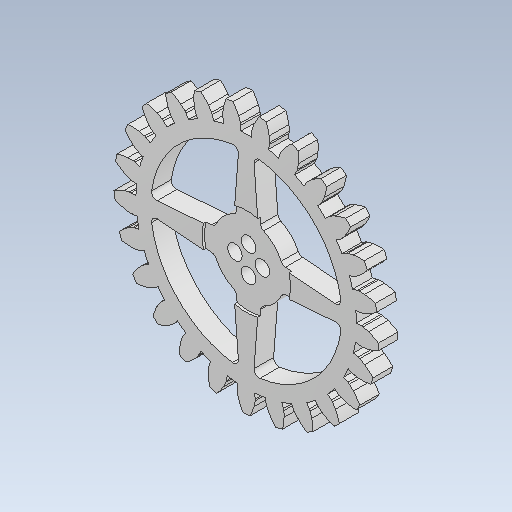
# Autodesk Inventor part: ｍ2歯数25ギアネジ
Saved by Autodesk Inventor 2020.2 (Build 242310000, 310)
## iProperties
Created: 2020-04-14
Part Number: ｍ2歯数25ギアネジ
Material: アルミニウム 2014-T4
Document SubType Name: Modeling
Designer: aoyama
Density: 2.8 g/cm^3
Appearance: サテン
Author: aoyama
Autodesk Inventor part; units mm, degrees
ref_plane "YZ Plane" through (0, 0, 0) normal (1, 0, 0) x (0, 1, 0)
ref_plane "XZ Plane" through (0, 0, 0) normal (0, 1, 0) x (-1, 0, 0)
ref_plane "XY Plane" through (0, 0, 0) normal (0, 0, 1) x (1, 0, 0)
sketch "スケッチ1" plane through (0, 0, 0) normal (0, 0, 1) x (1, 0, 0)
  arc A0 (-5.045, 28.8847) -> (-5.1025, 28.5361) centre (-2.8234, 28.3389) ccw
  arc A1 (-4.679, 29.9735) -> (-5.045, 28.8847) centre (1.0751, 27.4336) ccw
  arc A2 (-3.5593, 31.9385) -> (-4.679, 29.9735) centre (5.2754, 25.6027) ccw
  arc A3 (-7.3535, 28.5361) -> (-7.4111, 28.8847) centre (-9.6326, 28.3389) ccw
  arc A4 (-7.4111, 28.8847) -> (-7.777, 29.9735) centre (-13.5311, 27.4336) ccw
  arc A5 (-7.777, 29.9735) -> (-8.8968, 31.9385) centre (-17.7315, 25.6027) ccw
  arc A6 (-5.1501, 27.5449) -> (-7.306, 27.5449) centre (-6.228, 5.0707) ccw
  arc A7 (-8.8968, 31.9385) -> (-10.3249, 31.7581) centre (-6.228, 5.0707) ccw
  line L0 (-5.1501, 27.5449) -> (-5.1025, 28.5361)
  line L1 (-7.306, 27.5449) -> (-7.3535, 28.5361)
  arc A8 (-15.4947, 30.4307) -> (-16.8331, 29.9008) centre (-6.228, 5.0707) ccw
  arc A9 (-13.9214, 28.8059) -> (-15.4947, 30.4307) centre (-22.4762, 22.0969) ccw
  arc A10 (-13.2962, 27.8424) -> (-13.9214, 28.8059) centre (-18.8631, 24.9148) ccw
  line L2 (-12.8612, 26.5708) -> (-13.1538, 27.519)
  arc A11 (-13.1538, 27.519) -> (-13.2962, 27.8424) centre (-15.3122, 26.7612) ccw
  arc A12 (-11.0044, 28.4308) -> (-10.9735, 28.0788) centre (-8.7169, 28.4546) ccw
  arc A13 (-10.773, 27.1069) -> (-12.8612, 26.5708) centre (-6.228, 5.0707) ccw
  arc A14 (-10.9208, 29.5763) -> (-11.0044, 28.4308) centre (-4.7158, 28.5472) ccw
  arc A15 (-10.3249, 31.7581) -> (-10.9208, 29.5763) centre (-0.1921, 27.8185) ccw
  line L3 (-10.773, 27.1069) -> (-10.9735, 28.0788)
  arc A16 (-21.5103, 27.3295) -> (-22.6749, 26.4834) centre (-6.228, 5.0707) ccw
  arc A17 (-19.5824, 26.1469) -> (-21.5103, 27.3295) centre (-26.1999, 17.5212) ccw
  arc A18 (-18.7372, 25.3692) -> (-19.5824, 26.1469) centre (-23.4012, 21.1491) ccw
  line L4 (-17.9997, 24.2457) -> (-18.5188, 25.0914)
  arc A19 (-18.5188, 25.0914) -> (-18.7372, 25.3692) centre (-20.421, 23.8206) ccw
  arc A20 (-16.6638, 26.509) -> (-16.5463, 26.1758) centre (-14.4541, 27.101) ccw
  arc A21 (-16.1104, 25.2843) -> (-17.9997, 24.2457) centre (-6.228, 5.0707) ccw
  arc A22 (-16.8676, 27.6394) -> (-16.6638, 26.509) centre (-10.6017, 28.1857) ccw
  arc A23 (-16.8331, 29.9008) -> (-16.8676, 27.6394) centre (-6.0388, 28.6049) ccw
  line L5 (-16.1104, 25.2843) -> (-16.5463, 26.1758)
  arc A24 (-26.5657, 22.8296) -> (-27.4833, 21.7205) centre (-6.228, 5.0707) ccw
  arc A25 (-24.4043, 22.1637) -> (-26.5657, 22.8296) centre (-28.6688, 12.1633) ccw
  arc A26 (-23.3922, 21.6205) -> (-24.4043, 22.1637) centre (-26.8602, 16.3732) ccw
  line L6 (-22.3984, 20.7158) -> (-23.1116, 21.4058)
  arc A27 (-23.1116, 21.4058) -> (-23.3922, 21.6205) centre (-24.638, 19.7019) ccw
  arc A28 (-21.6674, 23.2402) -> (-21.4707, 22.9467) centre (-19.6743, 24.3631) ccw
  arc A29 (-20.8269, 22.1916) -> (-22.3984, 20.7158) centre (-6.228, 5.0707) ccw
  arc A30 (-22.146, 24.2844) -> (-21.6674, 23.2402) centre (-16.2127, 26.3719) ccw
  arc A31 (-22.6749, 26.4834) -> (-22.146, 24.2844) centre (-11.8975, 27.9126) ccw
  line L7 (-20.8269, 22.1916) -> (-21.4707, 22.9467)
  arc A32 (-30.3432, 17.2139) -> (-30.9561, 15.9115) centre (-6.228, 5.0707) ccw
  arc A33 (-28.0841, 17.1064) -> (-30.3432, 17.2139) centre (-29.7276, 6.3596) ccw
  arc A34 (-26.9688, 16.832) -> (-28.0841, 17.1064) centre (-29.0228, 10.8871) ccw
  line L8 (-25.7812, 16.2029) -> (-26.6435, 16.6938)
  arc A35 (-26.6435, 16.6938) -> (-26.9688, 16.832) centre (-27.6983, 14.6638) ccw
  arc A36 (-25.7009, 18.8298) -> (-25.4374, 18.5944) centre (-24.0497, 20.4131) ccw
  arc A37 (-24.626, 18.0232) -> (-25.7812, 16.2029) centre (-6.228, 5.0707) ccw
  arc A38 (-26.4241, 19.7222) -> (-25.7009, 18.8298) centre (-21.1964, 23.2196) ccw
  arc A39 (-27.4833, 21.7205) -> (-26.4241, 19.7222) centre (-17.3999, 25.785) ccw
  line L9 (-24.626, 18.0232) -> (-25.4374, 18.5944)
  arc A40 (-32.6055, 10.8352) -> (-32.8752, 9.4213) centre (-6.228, 5.0707) ccw
  arc A41 (-30.3906, 11.2929) -> (-32.6055, 10.8352) centre (-29.3099, 0.475) ccw
  arc A42 (-29.2421, 11.3045) -> (-30.3906, 11.2929) centre (-29.7531, 5.0356) ccw
  line L10 (-27.9353, 10.9904) -> (-28.8927, 11.2515)
  arc A43 (-28.8927, 11.2515) -> (-29.2421, 11.3045) centre (-29.4094, 9.023) ccw
  arc A44 (-28.5109, 13.5548) -> (-28.1971, 13.3923) centre (-27.3053, 15.499) ccw
  arc A45 (-27.2691, 13.0408) -> (-27.9353, 10.9904) centre (-6.228, 5.0707) ccw
  arc A46 (-29.4333, 14.2393) -> (-28.5109, 13.5548) centre (-25.2396, 18.9269) ccw
  arc A47 (-30.9561, 15.9115) -> (-29.4333, 14.2393) centre (-22.2003, 22.3559) ccw
  line L11 (-27.2691, 13.0408) -> (-28.1971, 13.3923)
  arc A48 (-33.2104, 4.0943) -> (-33.12, 2.6577) centre (-6.228, 5.0707) ccw
  arc A49 (-31.1789, 5.0885) -> (-33.2104, 4.0943) centre (-27.4418, -5.1208) ccw
  arc A50 (-30.0693, 5.3853) -> (-31.1789, 5.0885) centre (-29.0053, -0.8138) ccw
  line L12 (-28.7255, 5.4061) -> (-29.7177, 5.4209)
  arc A51 (-29.7177, 5.4209) -> (-30.0693, 5.3853) centre (-29.664, 3.1339) ccw
  arc A52 (-29.9207, 7.7468) -> (-29.5764, 7.6674) centre (-29.2365, 9.9297) ccw
  arc A53 (-28.5902, 7.5577) -> (-28.7255, 5.4061) centre (-6.228, 5.0707) ccw
  arc A54 (-30.9844, 8.1803) -> (-29.9207, 7.7468) centre (-28.0882, 13.7636) ccw
  arc A55 (-32.8752, 9.4213) -> (-30.9844, 8.1803) centre (-25.9972, 17.8407) ccw
  line L13 (-28.5902, 7.5577) -> (-29.5764, 7.6674)
  arc A56 (-32.1198, -2.5852) -> (-31.675, -3.9543) centre (-6.228, 5.0707) ccw
  arc A57 (-30.3994, -1.1171) -> (-32.1198, -2.5852) centre (-24.2408, -10.0763) ccw
  arc A58 (-29.3985, -0.5536) -> (-30.3994, -1.1171) centre (-26.8263, -6.2934) ccw
  line L14 (-28.1021, -0.1994) -> (-29.0668, -0.4318)
  arc A59 (-29.0668, -0.4318) -> (-29.3985, -0.5536) centre (-28.4461, -2.6336) ccw
  arc A60 (-29.8419, 1.7705) -> (-29.4886, 1.7793) centre (-29.722, 4.055) ccw
  arc A61 (-28.5061, 1.9184) -> (-28.1021, -0.1994) centre (-6.228, 5.0707) ccw
  arc A62 (-30.9799, 1.926) -> (-29.8419, 1.7705) centre (-29.5632, 8.0541) ccw
  arc A63 (-33.12, 2.6577) -> (-30.9799, 1.926) centre (-28.5519, 12.5231) ccw
  line L15 (-28.5061, 1.9184) -> (-29.4886, 1.7793)
  arc A64 (-29.4024, -8.7837) -> (-28.6311, -9.9991) centre (-6.228, 5.0707) ccw
  arc A65 (-28.1012, -6.9339) -> (-29.4024, -8.7837) centre (-19.908, -14.08) ccw
  arc A66 (-27.2718, -6.1392) -> (-28.1012, -6.9339) centre (-23.353, -11.0589) ccw
  line L16 (-26.1043, -5.4737) -> (-26.9809, -5.9387)
  arc A67 (-26.9809, -5.9387) -> (-27.2718, -6.1392) centre (-25.8321, -7.9169) ccw
  arc A68 (-28.2793, -3.9983) -> (-27.9393, -3.9019) centre (-28.7313, -1.7558) ccw
  arc A69 (-27.0222, -3.5229) -> (-26.1043, -5.4737) centre (-6.228, 5.0707) ccw
  arc A70 (-29.4202, -4.1308) -> (-28.2793, -3.9983) centre (-29.572, 2.1572) ccw
  arc A71 (-31.675, -3.9543) -> (-29.4202, -4.1308) centre (-29.7038, 6.7373) ccw
  line L17 (-27.0222, -3.5229) -> (-27.9393, -3.9019)
  arc A72 (-25.2289, -14.1117) -> (-24.1796, -15.0971) centre (-6.228, 5.0707) ccw
  arc A73 (-24.4285, -11.9964) -> (-25.2289, -14.1117) centre (-14.7156, -16.8804) ccw
  arc A74 (-23.8229, -11.0204) -> (-24.4285, -11.9964) centre (-18.8037, -14.811) ccw
  line L18 (-22.8576, -10.0854) -> (-23.591, -10.7538)
  arc A75 (-23.591, -10.7538) -> (-23.8229, -11.0204) centre (-21.9863, -12.3842) ccw
  arc A76 (-25.3311, -9.1973) -> (-25.0258, -9.0194) centre (-26.3266, -7.1376) ccw
  arc A77 (-24.2318, -8.4242) -> (-22.8576, -10.0854) centre (-6.228, 5.0707) ccw
  arc A78 (-26.4033, -9.6093) -> (-25.3311, -9.1973) centre (-28.1141, -3.5567) ccw
  arc A79 (-28.6311, -9.9991) -> (-26.4033, -9.6093) centre (-29.3808, 0.8467) ccw
  line L19 (-24.2318, -8.4242) -> (-25.0258, -9.0194)
  arc A80 (-19.8615, -18.2344) -> (-18.6, -18.9279) centre (-6.228, 5.0707) ccw
  arc A81 (-19.6123, -15.9865) -> (-19.8615, -18.2344) centre (-8.9899, -18.3015) ccw
  arc A82 (-19.2684, -14.8906) -> (-19.6123, -15.9865) centre (-13.4642, -17.3138) ccw
  line L20 (-18.5659, -13.7448) -> (-19.1101, -14.5747)
  arc A83 (-19.1101, -14.5747) -> (-19.2684, -14.8906) centre (-17.1503, -15.7548) ccw
  arc A84 (-21.1826, -13.4998) -> (-20.9312, -13.2516) centre (-22.6591, -11.7524) ccw
  arc A85 (-20.3101, -12.4776) -> (-18.5659, -13.7448) centre (-6.228, 5.0707) ccw
  arc A86 (-22.1186, -14.1655) -> (-21.1826, -13.4998) centre (-25.2809, -8.7285) ccw
  arc A87 (-24.1796, -15.0971) -> (-22.1186, -14.1655) centre (-27.6029, -4.7784) ccw
  line L21 (-20.3101, -12.4776) -> (-20.9312, -13.2516)
  arc A88 (-13.6374, -20.8927) -> (-12.2431, -21.2507) centre (-6.228, 5.0707) ccw
  arc A89 (-13.9551, -18.6534) -> (-13.6374, -20.8927) centre (-3.0907, -18.2541) ccw
  arc A90 (-13.8946, -17.5064) -> (-13.9551, -18.6534) centre (-7.6701, -18.4101) ccw
  line L22 (-13.4991, -16.222) -> (-13.8197, -17.1611)
  arc A91 (-13.8197, -17.1611) -> (-13.8946, -17.5064) centre (-11.6281, -17.8168) ccw
  arc A92 (-16.0945, -16.6354) -> (-15.9127, -16.3325) centre (-17.9591, -15.3101) ccw
  arc A93 (-15.5036, -15.4284) -> (-13.4991, -16.222) centre (-6.228, 5.0707) ccw
  arc A94 (-16.8356, -17.513) -> (-16.0945, -16.6354) centre (-21.2506, -13.0332) ccw
  arc A95 (-18.6, -18.9279) -> (-16.8356, -17.513) centre (-24.482, -9.7847) ccw
  line L23 (-15.5036, -15.4284) -> (-15.9127, -16.3325)
  arc A96 (-6.9478, -21.9197) -> (-5.5083, -21.9197) centre (-6.228, 5.0707) ccw
  arc A97 (-7.8124, -19.8298) -> (-6.9478, -21.9197) centre (2.6114, -16.7411) ccw
  arc A98 (-8.039, -18.7037) -> (-7.8124, -19.8298) centre (-1.7853, -18.0311) ccw
  line L24 (-7.9753, -17.3613) -> (-8.0524, -18.3506)
  arc A99 (-8.0524, -18.3506) -> (-8.039, -18.7037) centre (-5.7665, -18.4406) ccw
  arc A100 (-10.3864, -18.4072) -> (-10.2856, -18.0685) centre (-12.5221, -17.5872) ccw
  arc A101 (-10.1142, -17.0911) -> (-7.9753, -17.3613) centre (-6.228, 5.0707) ccw
  arc A102 (-10.8859, -19.4415) -> (-10.3864, -18.4072) centre (-16.2763, -16.2004) ccw
  arc A103 (-12.2431, -21.2507) -> (-10.8859, -19.4415) centre (-20.2141, -13.8576) ccw
  line L25 (-10.1142, -17.0911) -> (-10.2856, -18.0685)
  arc A104 (-0.2129, -21.2507) -> (1.1813, -20.8927) centre (-6.228, 5.0707) ccw
  arc A105 (-1.5701, -19.4415) -> (-0.2129, -21.2507) centre (7.758, -13.8576) ccw
  arc A106 (-2.0696, -18.4072) -> (-1.5701, -19.4415) centre (3.8203, -16.2004) ccw
  line L26 (-2.3418, -17.0911) -> (-2.1704, -18.0685)
  arc A107 (-2.1704, -18.0685) -> (-2.0696, -18.4072) centre (0.066, -17.5872) ccw
  arc A108 (-4.4171, -18.7037) -> (-4.4037, -18.3506) centre (-6.6895, -18.4406) ccw
  arc A109 (-4.4807, -17.3613) -> (-2.3418, -17.0911) centre (-6.228, 5.0707) ccw
  arc A110 (-4.6437, -19.8298) -> (-4.4171, -18.7037) centre (-10.6707, -18.0311) ccw
  arc A111 (-5.5083, -21.9197) -> (-4.6437, -19.8298) centre (-15.0674, -16.7411) ccw
  line L27 (-4.4807, -17.3613) -> (-4.4037, -18.3506)
  arc A112 (6.144, -18.9279) -> (7.4054, -18.2344) centre (-6.228, 5.0707) ccw
  arc A113 (4.3795, -17.513) -> (6.144, -18.9279) centre (12.0259, -9.7847) ccw
  arc A114 (3.6385, -16.6354) -> (4.3795, -17.513) centre (8.7945, -13.0332) ccw
  line L28 (3.0475, -15.4284) -> (3.4566, -16.3325)
  arc A115 (3.4566, -16.3325) -> (3.6385, -16.6354) centre (5.5031, -15.3101) ccw
  arc A116 (1.4385, -17.5064) -> (1.3637, -17.1611) centre (-0.828, -17.8168) ccw
  arc A117 (1.043, -16.222) -> (3.0475, -15.4284) centre (-6.228, 5.0707) ccw
  arc A118 (1.4991, -18.6534) -> (1.4385, -17.5064) centre (-4.786, -18.4101) ccw
  arc A119 (1.1813, -20.8927) -> (1.4991, -18.6534) centre (-9.3653, -18.2541) ccw
  line L29 (1.043, -16.222) -> (1.3637, -17.1611)
  arc A120 (11.7235, -15.0971) -> (12.7728, -14.1117) centre (-6.228, 5.0707) ccw
  arc A121 (9.6626, -14.1655) -> (11.7235, -15.0971) centre (15.1468, -4.7784) ccw
  arc A122 (8.7266, -13.4998) -> (9.6626, -14.1655) centre (12.8248, -8.7285) ccw
  line L30 (7.854, -12.4776) -> (8.4751, -13.2516)
  arc A123 (8.4751, -13.2516) -> (8.7266, -13.4998) centre (10.203, -11.7524) ccw
  arc A124 (6.8124, -14.8906) -> (6.654, -14.5747) centre (4.6943, -15.7548) ccw
  arc A125 (6.1099, -13.7448) -> (7.854, -12.4776) centre (-6.228, 5.0707) ccw
  arc A126 (7.1563, -15.9865) -> (6.8124, -14.8906) centre (1.0082, -17.3138) ccw
  arc A127 (7.4054, -18.2344) -> (7.1563, -15.9865) centre (-3.4661, -18.3015) ccw
  line L31 (6.1099, -13.7448) -> (6.654, -14.5747)
  arc A128 (16.1751, -9.9991) -> (16.9464, -8.7837) centre (-6.228, 5.0707) ccw
  arc A129 (13.9472, -9.6093) -> (16.1751, -9.9991) centre (16.9247, 0.8467) ccw
  arc A130 (12.8751, -9.1973) -> (13.9472, -9.6093) centre (15.658, -3.5567) ccw
  line L32 (11.7757, -8.4242) -> (12.5697, -9.0194)
  arc A131 (12.5697, -9.0194) -> (12.8751, -9.1973) centre (13.8706, -7.1376) ccw
  arc A132 (11.3669, -11.0204) -> (11.1349, -10.7538) centre (9.5302, -12.3842) ccw
  arc A133 (10.4015, -10.0854) -> (11.7757, -8.4242) centre (-6.228, 5.0707) ccw
  arc A134 (11.9725, -11.9964) -> (11.3669, -11.0204) centre (6.3477, -14.811) ccw
  arc A135 (12.7728, -14.1117) -> (11.9725, -11.9964) centre (2.2596, -16.8804) ccw
  line L33 (10.4015, -10.0854) -> (11.1349, -10.7538)
  arc A136 (19.219, -3.9543) -> (19.6638, -2.5852) centre (-6.228, 5.0707) ccw
  arc A137 (16.9642, -4.1308) -> (19.219, -3.9543) centre (17.2478, 6.7373) ccw
  arc A138 (15.8232, -3.9983) -> (16.9642, -4.1308) centre (17.116, 2.1572) ccw
  line L34 (14.5662, -3.5229) -> (15.4833, -3.9019)
  arc A139 (15.4833, -3.9019) -> (15.8232, -3.9983) centre (16.2752, -1.7558) ccw
  arc A140 (14.8158, -6.1392) -> (14.5248, -5.9387) centre (13.376, -7.9169) ccw
  arc A141 (13.6482, -5.4737) -> (14.5662, -3.5229) centre (-6.228, 5.0707) ccw
  arc A142 (15.6451, -6.9339) -> (14.8158, -6.1392) centre (10.897, -11.0589) ccw
  arc A143 (16.9464, -8.7837) -> (15.6451, -6.9339) centre (7.4519, -14.08) ccw
  line L35 (13.6482, -5.4737) -> (14.5248, -5.9387)
  arc A144 (20.6639, 2.6577) -> (20.7543, 4.0943) centre (-6.228, 5.0707) ccw
  arc A145 (18.5239, 1.926) -> (20.6639, 2.6577) centre (16.0958, 12.5231) ccw
  arc A146 (17.3858, 1.7705) -> (18.5239, 1.926) centre (17.1072, 8.0541) ccw
  line L36 (16.05, 1.9184) -> (17.0326, 1.7793)
  arc A147 (17.0326, 1.7793) -> (17.3858, 1.7705) centre (17.2659, 4.055) ccw
  arc A148 (16.9425, -0.5536) -> (16.6108, -0.4318) centre (15.99, -2.6336) ccw
  arc A149 (15.6461, -0.1994) -> (16.05, 1.9184) centre (-6.228, 5.0707) ccw
  arc A150 (17.9433, -1.1171) -> (16.9425, -0.5536) centre (14.3702, -6.2934) ccw
  arc A151 (19.6638, -2.5852) -> (17.9433, -1.1171) centre (11.7847, -10.0763) ccw
  line L37 (15.6461, -0.1994) -> (16.6108, -0.4318)
  arc A152 (20.4192, 9.4213) -> (20.1494, 10.8352) centre (-6.228, 5.0707) ccw
  arc A153 (18.5283, 8.1803) -> (20.4192, 9.4213) centre (13.5411, 17.8407) ccw
  arc A154 (17.4647, 7.7468) -> (18.5283, 8.1803) centre (15.6321, 13.7636) ccw
  line L38 (16.1341, 7.5577) -> (17.1203, 7.6674)
  arc A155 (17.1203, 7.6674) -> (17.4647, 7.7468) centre (16.7804, 9.9297) ccw
  arc A156 (17.6132, 5.3853) -> (17.2617, 5.4209) centre (17.208, 3.1339) ccw
  arc A157 (16.2695, 5.4061) -> (16.1341, 7.5577) centre (-6.228, 5.0707) ccw
  arc A158 (18.7228, 5.0885) -> (17.6132, 5.3853) centre (16.5492, -0.8138) ccw
  arc A159 (20.7543, 4.0943) -> (18.7228, 5.0885) centre (14.9857, -5.1208) ccw
  line L39 (16.2695, 5.4061) -> (17.2617, 5.4209)
  arc A160 (18.5001, 15.9115) -> (17.8872, 17.2139) centre (-6.228, 5.0707) ccw
  arc A161 (16.9772, 14.2393) -> (18.5001, 15.9115) centre (9.7443, 22.3559) ccw
  arc A162 (16.0548, 13.5548) -> (16.9772, 14.2393) centre (12.7835, 18.9269) ccw
  line L40 (14.8131, 13.0408) -> (15.741, 13.3923)
  arc A163 (15.741, 13.3923) -> (16.0548, 13.5548) centre (14.8492, 15.499) ccw
  arc A164 (16.786, 11.3045) -> (16.4366, 11.2515) centre (16.9534, 9.023) ccw
  arc A165 (15.4793, 10.9904) -> (14.8131, 13.0408) centre (-6.228, 5.0707) ccw
  arc A166 (17.9345, 11.2929) -> (16.786, 11.3045) centre (17.2971, 5.0356) ccw
  arc A167 (20.1494, 10.8352) -> (17.9345, 11.2929) centre (16.8538, 0.475) ccw
  line L41 (15.4793, 10.9904) -> (16.4366, 11.2515)
  arc A168 (15.0272, 21.7205) -> (14.1097, 22.8296) centre (-6.228, 5.0707) ccw
  arc A169 (13.968, 19.7222) -> (15.0272, 21.7205) centre (4.9438, 25.785) ccw
  arc A170 (13.2449, 18.8298) -> (13.968, 19.7222) centre (8.7403, 23.2196) ccw
  line L42 (12.1699, 18.0232) -> (12.9813, 18.5944)
  arc A171 (12.9813, 18.5944) -> (13.2449, 18.8298) centre (11.5936, 20.4131) ccw
  arc A172 (14.5127, 16.832) -> (14.1875, 16.6938) centre (15.2422, 14.6638) ccw
  arc A173 (13.3251, 16.2029) -> (12.1699, 18.0232) centre (-6.228, 5.0707) ccw
  arc A174 (15.628, 17.1064) -> (14.5127, 16.832) centre (16.5667, 10.8871) ccw
  arc A175 (17.8872, 17.2139) -> (15.628, 17.1064) centre (17.2715, 6.3596) ccw
  line L43 (13.3251, 16.2029) -> (14.1875, 16.6938)
  arc A176 (10.2188, 26.4834) -> (9.0543, 27.3295) centre (-6.228, 5.0707) ccw
  arc A177 (9.6899, 24.2844) -> (10.2188, 26.4834) centre (-0.5586, 27.9126) ccw
  arc A178 (9.2114, 23.2402) -> (9.6899, 24.2844) centre (3.7567, 26.3719) ccw
  line L44 (8.3708, 22.1916) -> (9.0146, 22.9467)
  arc A179 (9.0146, 22.9467) -> (9.2114, 23.2402) centre (7.2183, 24.3631) ccw
  arc A180 (10.9362, 21.6205) -> (10.6556, 21.4058) centre (12.182, 19.7019) ccw
  arc A181 (9.9424, 20.7158) -> (8.3708, 22.1916) centre (-6.228, 5.0707) ccw
  arc A182 (11.9482, 22.1637) -> (10.9362, 21.6205) centre (14.4041, 16.3732) ccw
  arc A183 (14.1097, 22.8296) -> (11.9482, 22.1637) centre (16.2127, 12.1633) ccw
  line L45 (9.9424, 20.7158) -> (10.6556, 21.4058)
  arc A184 (4.377, 29.9008) -> (3.0386, 30.4307) centre (-6.228, 5.0707) ccw
  arc A185 (4.4116, 27.6394) -> (4.377, 29.9008) centre (-6.4172, 28.6049) ccw
  arc A186 (4.2077, 26.509) -> (4.4116, 27.6394) centre (-1.8544, 28.1857) ccw
  line L46 (3.6544, 25.2843) -> (4.0902, 26.1758)
  arc A187 (4.0902, 26.1758) -> (4.2077, 26.509) centre (1.998, 27.101) ccw
  arc A188 (6.2812, 25.3692) -> (6.0628, 25.0914) centre (7.965, 23.8206) ccw
  arc A189 (5.5436, 24.2457) -> (3.6544, 25.2843) centre (-6.228, 5.0707) ccw
  arc A190 (7.1263, 26.1469) -> (6.2812, 25.3692) centre (10.9451, 21.1491) ccw
  arc A191 (9.0543, 27.3295) -> (7.1263, 26.1469) centre (13.7439, 17.5212) ccw
  line L47 (5.5436, 24.2457) -> (6.0628, 25.0914)
  arc A192 (-2.1312, 31.7581) -> (-3.5593, 31.9385) centre (-6.228, 5.0707) ccw
  arc A193 (-1.5353, 29.5763) -> (-2.1312, 31.7581) centre (-12.264, 27.8185) ccw
  arc A194 (-1.4516, 28.4308) -> (-1.5353, 29.5763) centre (-7.7403, 28.5472) ccw
  line L48 (-1.683, 27.1069) -> (-1.4826, 28.0788)
  arc A195 (-1.4826, 28.0788) -> (-1.4516, 28.4308) centre (-3.7391, 28.4546) ccw
  arc A196 (0.8402, 27.8424) -> (0.6977, 27.519) centre (2.8562, 26.7612) ccw
  arc A197 (0.4052, 26.5708) -> (-1.683, 27.1069) centre (-6.228, 5.0707) ccw
  arc A198 (1.4654, 28.8059) -> (0.8402, 27.8424) centre (6.407, 24.9148) ccw
  arc A199 (3.0386, 30.4307) -> (1.4654, 28.8059) centre (10.0201, 22.0969) ccw
  line L49 (0.4052, 26.5708) -> (0.6977, 27.519)
  line L50 (-6.228, 5.0707) -> (-6.228, 7.8707) construction
  circle A200 centre (-6.228, 7.8707) radius 2.8 construction
  circle A201 centre (-9.028, 5.0707) radius 2.8 construction
  circle A202 centre (-6.228, 2.2707) radius 2.8 construction
  circle A203 centre (-3.428, 5.0707) radius 2.8 construction
  circle A204 centre (-6.228, 7.8707) radius 1.5
  circle A205 centre (-9.028, 5.0707) radius 1.5
  circle A206 centre (-6.228, 2.2707) radius 1.5
  circle A207 centre (-3.428, 5.0707) radius 1.5
  point P0 (0, 0)
  point P1 (3.4566, -16.3325)
  point P2 (3.6385, -16.6354)
  point P3 (4.3795, -17.513)
  point P4 (6.144, -18.9279)
  point P5 (7.4054, -18.2344)
  point P6 (7.1563, -15.9865)
  point P7 (6.8124, -14.8906)
  point P8 (7.854, -12.4776)
  point P9 (8.4751, -13.2516)
  point P10 (8.7266, -13.4998)
  point P11 (9.6626, -14.1655)
  point P12 (11.7235, -15.0971)
  point P13 (12.7728, -14.1117)
  point P14 (11.9725, -11.9964)
  point P15 (11.3669, -11.0204)
  point P16 (11.7757, -8.4242)
  point P17 (12.5697, -9.0194)
  point P18 (12.8751, -9.1973)
  point P19 (13.9472, -9.6093)
  point P20 (16.1751, -9.9991)
  point P21 (16.9464, -8.7837)
  point P22 (15.6451, -6.9339)
  point P23 (14.8158, -6.1392)
  point P24 (14.5662, -3.5229)
  point P25 (15.4833, -3.9019)
  point P26 (15.8232, -3.9983)
  point P27 (16.9642, -4.1308)
  point P28 (19.219, -3.9543)
  point P29 (19.6638, -2.5852)
  point P30 (17.9433, -1.1171)
  point P31 (16.9425, -0.5536)
  point P32 (16.05, 1.9184)
  point P33 (17.0326, 1.7793)
  point P34 (17.3858, 1.7705)
  point P35 (18.5239, 1.926)
  point P36 (20.6639, 2.6577)
  point P37 (20.7543, 4.0943)
  point P38 (18.7228, 5.0885)
  point P39 (17.6132, 5.3853)
  point P40 (16.1341, 7.5577)
  point P41 (17.1203, 7.6674)
  point P42 (17.4647, 7.7468)
  point P43 (18.5283, 8.1803)
  point P44 (20.4192, 9.4213)
  point P45 (20.1494, 10.8352)
  point P46 (17.9345, 11.2929)
  point P47 (16.786, 11.3045)
  point P48 (14.8131, 13.0408)
  point P49 (15.741, 13.3923)
  point P50 (16.0548, 13.5548)
  point P51 (16.9772, 14.2393)
  point P52 (18.5001, 15.9115)
  point P53 (17.8872, 17.2139)
  point P54 (15.628, 17.1064)
  point P55 (14.5127, 16.832)
  point P56 (12.1699, 18.0232)
  point P57 (12.9813, 18.5944)
  point P58 (13.2449, 18.8298)
  point P59 (13.968, 19.7222)
  point P60 (15.0272, 21.7205)
  point P61 (14.1097, 22.8296)
  point P62 (11.9482, 22.1637)
  point P63 (10.9362, 21.6205)
  point P64 (8.3708, 22.1916)
  point P65 (9.0146, 22.9467)
  point P66 (9.2114, 23.2402)
  point P67 (9.6899, 24.2844)
  point P68 (10.2188, 26.4834)
  point P69 (9.0543, 27.3295)
  point P70 (7.1263, 26.1469)
  point P71 (6.2812, 25.3692)
  point P72 (3.6544, 25.2843)
  point P73 (4.0902, 26.1758)
  point P74 (4.2077, 26.509)
  point P75 (4.4116, 27.6394)
  point P76 (4.377, 29.9008)
  point P77 (3.0386, 30.4307)
  point P78 (1.4654, 28.8059)
  point P79 (0.8402, 27.8424)
  point P80 (-1.683, 27.1069)
  point P81 (-1.4826, 28.0788)
  point P82 (-1.4516, 28.4308)
  point P83 (-1.5353, 29.5763)
  point P84 (-2.1312, 31.7581)
  point P85 (-3.5593, 31.9385)
  point P86 (-4.679, 29.9735)
  point P87 (-5.045, 28.8847)
  point P88 (-7.4111, 28.8847)
  point P89 (-7.777, 29.9735)
  point P90 (-8.8968, 31.9385)
  point P91 (-10.3249, 31.7581)
  point P92 (-10.9208, 29.5763)
  point P93 (-11.0044, 28.4308)
  point P94 (-12.8612, 26.5708)
  point P95 (-13.1538, 27.519)
  point P96 (-13.2962, 27.8424)
  point P97 (-13.9214, 28.8059)
  point P98 (-15.4947, 30.4307)
  point P99 (-16.8331, 29.9008)
  point P100 (-16.8676, 27.6394)
  point P101 (-16.6638, 26.509)
  point P102 (-17.9997, 24.2457)
  point P103 (-18.5188, 25.0914)
  point P104 (-18.7372, 25.3692)
  point P105 (-19.5824, 26.1469)
  point P106 (-22.6749, 26.4834)
  point P107 (-22.146, 24.2844)
  point P108 (-21.6674, 23.2402)
  point P109 (-22.3984, 20.7158)
  point P110 (-23.1116, 21.4058)
  point P111 (-23.3922, 21.6205)
  point P112 (-24.4043, 22.1637)
  point P113 (-26.5657, 22.8296)
  point P114 (-27.4833, 21.7205)
  point P115 (-26.4241, 19.7222)
  point P116 (-25.7009, 18.8298)
  point P117 (-25.7812, 16.2029)
  point P118 (-26.6435, 16.6938)
  point P119 (-26.9688, 16.832)
  point P120 (-28.0841, 17.1064)
  point P121 (-30.3432, 17.2139)
  point P122 (-30.9561, 15.9115)
  point P123 (-29.4333, 14.2393)
  point P124 (-28.5109, 13.5548)
  point P125 (-27.9353, 10.9904)
  point P126 (-28.8927, 11.2515)
  point P127 (-29.2421, 11.3045)
  point P128 (-30.3906, 11.2929)
  point P129 (-32.6055, 10.8352)
  point P130 (-32.8752, 9.4213)
  point P131 (-30.9844, 8.1803)
  point P132 (-29.9207, 7.7468)
  point P133 (-28.7255, 5.4061)
  point P134 (-29.7177, 5.4209)
  point P135 (-30.0693, 5.3853)
  point P136 (-31.1789, 5.0885)
  point P137 (-33.2104, 4.0943)
  point P138 (-33.12, 2.6577)
  point P139 (-30.9799, 1.926)
  point P140 (-29.8419, 1.7705)
  point P141 (-28.1021, -0.1994)
  point P142 (-29.0668, -0.4318)
  point P143 (-29.3985, -0.5536)
  point P144 (-30.3994, -1.1171)
  point P145 (-32.1198, -2.5852)
  point P146 (-31.675, -3.9543)
  point P147 (-29.4202, -4.1308)
  point P148 (-28.2793, -3.9983)
  point P149 (-26.1043, -5.4737)
  point P150 (-26.9809, -5.9387)
  point P151 (-27.2718, -6.1392)
  point P152 (-28.1012, -6.9339)
  point P153 (-29.4024, -8.7837)
  point P154 (-28.6311, -9.9991)
  point P155 (-26.4033, -9.6093)
  point P156 (-25.3311, -9.1973)
  point P157 (-22.8576, -10.0854)
  point P158 (-23.591, -10.7538)
  point P159 (-23.8229, -11.0204)
  point P160 (-24.4285, -11.9964)
  point P161 (-25.2289, -14.1117)
  point P162 (-24.1796, -15.0971)
  point P163 (-22.1186, -14.1655)
  point P164 (-21.1826, -13.4998)
  point P165 (-18.5659, -13.7448)
  point P166 (-19.1101, -14.5747)
  point P167 (-19.2684, -14.8906)
  point P168 (-19.6123, -15.9865)
  point P169 (-19.8615, -18.2344)
  point P170 (-18.6, -18.9279)
  point P171 (-16.8356, -17.513)
  point P172 (-16.0945, -16.6354)
  point P173 (-13.4991, -16.222)
  point P174 (-13.8197, -17.1611)
  point P175 (-13.8946, -17.5064)
  point P176 (-13.9551, -18.6534)
  point P177 (-13.6374, -20.8927)
  point P178 (-12.2431, -21.2507)
  point P179 (-10.8859, -19.4415)
  point P180 (-7.9753, -17.3613)
  point P181 (-8.0524, -18.3506)
  point P182 (-8.039, -18.7037)
  point P183 (-7.8124, -19.8298)
  point P184 (-6.9478, -21.9197)
  point P185 (-5.5083, -21.9197)
  point P186 (-4.6437, -19.8298)
  point P187 (-4.4171, -18.7037)
  point P188 (-2.3418, -17.0911)
  point P189 (-2.1704, -18.0685)
  point P190 (-2.0696, -18.4072)
  point P191 (-1.5701, -19.4415)
  point P192 (-0.2129, -21.2507)
  point P193 (1.1813, -20.8927)
  point P194 (1.4991, -18.6534)
  point P195 (1.4385, -17.5064)
  dimension "d2" = 360
  dimension "d4" = 5.6
  dimension "d7" = 360
  dimension "d9" = 3
  dimension "d12" = 360
  constraints: 400 point on circle, 208 centre point, 102 end point, 5 coincident, 1 equal radius, 1 vertical, 1005 other
  measures "d4" diameter of A200
  measures "d9" diameter of A204
extrude "押し出し1" add sketch "スケッチ1" along normal blind 4
sketch "スケッチ2" plane through (0, 0, 4) normal (0, 0, 1) x (1, 0, 0)
  arc A0 (12.7728, -14.1117) -> (11.9725, -11.9964) centre (2.2596, -16.8804) ccw projected
  arc A1 (11.9725, -11.9964) -> (11.3669, -11.0204) centre (6.3477, -14.811) ccw projected
  arc A2 (11.3669, -11.0204) -> (11.1349, -10.7538) centre (9.5302, -12.3842) ccw projected
  line L0 (11.1349, -10.7538) -> (10.4015, -10.0854) projected
  arc A3 (10.4015, -10.0854) -> (11.7757, -8.4242) centre (-6.228, 5.0707) ccw projected
  line L1 (11.7757, -8.4242) -> (12.5697, -9.0194) projected
  arc A4 (12.5697, -9.0194) -> (12.8751, -9.1973) centre (13.8706, -7.1376) ccw projected
  arc A5 (12.8751, -9.1973) -> (13.9472, -9.6093) centre (15.658, -3.5567) ccw projected
  arc A6 (13.9472, -9.6093) -> (16.1751, -9.9991) centre (16.9247, 0.8467) ccw projected
  arc A7 (16.1751, -9.9991) -> (16.9464, -8.7837) centre (-6.228, 5.0707) ccw projected
  arc A8 (16.9464, -8.7837) -> (15.6451, -6.9339) centre (7.4519, -14.08) ccw projected
  arc A9 (15.6451, -6.9339) -> (14.8158, -6.1392) centre (10.897, -11.0589) ccw projected
  arc A10 (14.8158, -6.1392) -> (14.5248, -5.9387) centre (13.376, -7.9169) ccw projected
  line L2 (14.5248, -5.9387) -> (13.6482, -5.4737) projected
  arc A11 (13.6482, -5.4737) -> (14.5662, -3.5229) centre (-6.228, 5.0707) ccw projected
  line L3 (14.5662, -3.5229) -> (15.4833, -3.9019) projected
  arc A12 (15.4833, -3.9019) -> (15.8232, -3.9983) centre (16.2752, -1.7558) ccw projected
  arc A13 (15.8232, -3.9983) -> (16.9642, -4.1308) centre (17.116, 2.1572) ccw projected
  arc A14 (16.9642, -4.1308) -> (19.219, -3.9543) centre (17.2478, 6.7373) ccw projected
  arc A15 (19.219, -3.9543) -> (19.6638, -2.5852) centre (-6.228, 5.0707) ccw projected
  arc A16 (19.6638, -2.5852) -> (17.9433, -1.1171) centre (11.7847, -10.0763) ccw projected
  arc A17 (17.9433, -1.1171) -> (16.9425, -0.5536) centre (14.3702, -6.2934) ccw projected
  arc A18 (16.9425, -0.5536) -> (16.6108, -0.4318) centre (15.99, -2.6336) ccw projected
  line L4 (16.6108, -0.4318) -> (15.6461, -0.1994) projected
  arc A19 (15.6461, -0.1994) -> (16.05, 1.9184) centre (-6.228, 5.0707) ccw projected
  line L5 (16.05, 1.9184) -> (17.0326, 1.7793) projected
  arc A20 (17.0326, 1.7793) -> (17.3858, 1.7705) centre (17.2659, 4.055) ccw projected
  arc A21 (17.3858, 1.7705) -> (18.5239, 1.926) centre (17.1072, 8.0541) ccw projected
  arc A22 (18.5239, 1.926) -> (20.6639, 2.6577) centre (16.0958, 12.5231) ccw projected
  arc A23 (20.6639, 2.6577) -> (20.7543, 4.0943) centre (-6.228, 5.0707) ccw projected
  arc A24 (20.7543, 4.0943) -> (18.7228, 5.0885) centre (14.9857, -5.1208) ccw projected
  arc A25 (18.7228, 5.0885) -> (17.6132, 5.3853) centre (16.5492, -0.8138) ccw projected
  arc A26 (17.6132, 5.3853) -> (17.2617, 5.4209) centre (17.208, 3.1339) ccw projected
  line L6 (17.2617, 5.4209) -> (16.2695, 5.4061) projected
  arc A27 (16.2695, 5.4061) -> (16.1341, 7.5577) centre (-6.228, 5.0707) ccw projected
  line L7 (16.1341, 7.5577) -> (17.1203, 7.6674) projected
  arc A28 (17.1203, 7.6674) -> (17.4647, 7.7468) centre (16.7804, 9.9297) ccw projected
  arc A29 (17.4647, 7.7468) -> (18.5283, 8.1803) centre (15.6321, 13.7636) ccw projected
  arc A30 (18.5283, 8.1803) -> (20.4192, 9.4213) centre (13.5411, 17.8407) ccw projected
  arc A31 (20.4192, 9.4213) -> (20.1494, 10.8352) centre (-6.228, 5.0707) ccw projected
  arc A32 (20.1494, 10.8352) -> (17.9345, 11.2929) centre (16.8538, 0.475) ccw projected
  arc A33 (17.9345, 11.2929) -> (16.786, 11.3045) centre (17.2971, 5.0356) ccw projected
  arc A34 (16.786, 11.3045) -> (16.4366, 11.2515) centre (16.9534, 9.023) ccw projected
  line L8 (16.4366, 11.2515) -> (15.4793, 10.9904) projected
  arc A35 (15.4793, 10.9904) -> (14.8131, 13.0408) centre (-6.228, 5.0707) ccw projected
  line L9 (14.8131, 13.0408) -> (15.741, 13.3923) projected
  arc A36 (15.741, 13.3923) -> (16.0548, 13.5548) centre (14.8492, 15.499) ccw projected
  arc A37 (16.0548, 13.5548) -> (16.9772, 14.2393) centre (12.7835, 18.9269) ccw projected
  arc A38 (16.9772, 14.2393) -> (18.5001, 15.9115) centre (9.7443, 22.3559) ccw projected
  arc A39 (18.5001, 15.9115) -> (17.8872, 17.2139) centre (-6.228, 5.0707) ccw projected
  arc A40 (17.8872, 17.2139) -> (15.628, 17.1064) centre (17.2715, 6.3596) ccw projected
  arc A41 (15.628, 17.1064) -> (14.5127, 16.832) centre (16.5667, 10.8871) ccw projected
  arc A42 (14.5127, 16.832) -> (14.1875, 16.6938) centre (15.2422, 14.6638) ccw projected
  line L10 (14.1875, 16.6938) -> (13.3251, 16.2029) projected
  arc A43 (13.3251, 16.2029) -> (12.1699, 18.0232) centre (-6.228, 5.0707) ccw projected
  line L11 (12.1699, 18.0232) -> (12.9813, 18.5944) projected
  arc A44 (12.9813, 18.5944) -> (13.2449, 18.8298) centre (11.5936, 20.4131) ccw projected
  arc A45 (13.2449, 18.8298) -> (13.968, 19.7222) centre (8.7403, 23.2196) ccw projected
  arc A46 (13.968, 19.7222) -> (15.0272, 21.7205) centre (4.9438, 25.785) ccw projected
  arc A47 (15.0272, 21.7205) -> (14.1097, 22.8296) centre (-6.228, 5.0707) ccw projected
  arc A48 (14.1097, 22.8296) -> (11.9482, 22.1637) centre (16.2127, 12.1633) ccw projected
  arc A49 (11.9482, 22.1637) -> (10.9362, 21.6205) centre (14.4041, 16.3732) ccw projected
  arc A50 (10.9362, 21.6205) -> (10.6556, 21.4058) centre (12.182, 19.7019) ccw projected
  line L12 (10.6556, 21.4058) -> (9.9424, 20.7158) projected
  arc A51 (9.9424, 20.7158) -> (8.3708, 22.1916) centre (-6.228, 5.0707) ccw projected
  line L13 (8.3708, 22.1916) -> (9.0146, 22.9467) projected
  arc A52 (9.0146, 22.9467) -> (9.2114, 23.2402) centre (7.2183, 24.3631) ccw projected
  arc A53 (9.2114, 23.2402) -> (9.6899, 24.2844) centre (3.7567, 26.3719) ccw projected
  arc A54 (9.6899, 24.2844) -> (10.2188, 26.4834) centre (-0.5586, 27.9126) ccw projected
  arc A55 (10.2188, 26.4834) -> (9.0543, 27.3295) centre (-6.228, 5.0707) ccw projected
  arc A56 (9.0543, 27.3295) -> (7.1263, 26.1469) centre (13.7439, 17.5212) ccw projected
  arc A57 (7.1263, 26.1469) -> (6.2812, 25.3692) centre (10.9451, 21.1491) ccw projected
  arc A58 (6.2812, 25.3692) -> (6.0628, 25.0914) centre (7.965, 23.8206) ccw projected
  line L14 (6.0628, 25.0914) -> (5.5436, 24.2457) projected
  arc A59 (5.5436, 24.2457) -> (3.6544, 25.2843) centre (-6.228, 5.0707) ccw projected
  line L15 (3.6544, 25.2843) -> (4.0902, 26.1758) projected
  arc A60 (4.0902, 26.1758) -> (4.2077, 26.509) centre (1.998, 27.101) ccw projected
  arc A61 (4.2077, 26.509) -> (4.4116, 27.6394) centre (-1.8544, 28.1857) ccw projected
  arc A62 (4.4116, 27.6394) -> (4.377, 29.9008) centre (-6.4172, 28.6049) ccw projected
  arc A63 (4.377, 29.9008) -> (3.0386, 30.4307) centre (-6.228, 5.0707) ccw projected
  arc A64 (3.0386, 30.4307) -> (1.4654, 28.8059) centre (10.0201, 22.0969) ccw projected
  arc A65 (1.4654, 28.8059) -> (0.8402, 27.8424) centre (6.407, 24.9148) ccw projected
  arc A66 (0.8402, 27.8424) -> (0.6977, 27.519) centre (2.8562, 26.7612) ccw projected
  line L16 (0.6977, 27.519) -> (0.4052, 26.5708) projected
  arc A67 (0.4052, 26.5708) -> (-1.683, 27.1069) centre (-6.228, 5.0707) ccw projected
  line L17 (-1.683, 27.1069) -> (-1.4826, 28.0788) projected
  arc A68 (-1.4826, 28.0788) -> (-1.4516, 28.4308) centre (-3.7391, 28.4546) ccw projected
  arc A69 (-1.4516, 28.4308) -> (-1.5353, 29.5763) centre (-7.7403, 28.5472) ccw projected
  arc A70 (-1.5353, 29.5763) -> (-2.1312, 31.7581) centre (-12.264, 27.8185) ccw projected
  arc A71 (-2.1312, 31.7581) -> (-3.5593, 31.9385) centre (-6.228, 5.0707) ccw projected
  arc A72 (-3.5593, 31.9385) -> (-4.679, 29.9735) centre (5.2754, 25.6027) ccw projected
  arc A73 (-4.679, 29.9735) -> (-5.045, 28.8847) centre (1.0751, 27.4336) ccw projected
  arc A74 (-5.045, 28.8847) -> (-5.1025, 28.5361) centre (-2.8234, 28.3389) ccw projected
  line L18 (-5.1025, 28.5361) -> (-5.1501, 27.5449) projected
  arc A75 (-5.1501, 27.5449) -> (-7.306, 27.5449) centre (-6.228, 5.0707) ccw projected
  line L19 (-7.306, 27.5449) -> (-7.3535, 28.5361) projected
  arc A76 (-7.3535, 28.5361) -> (-7.4111, 28.8847) centre (-9.6326, 28.3389) ccw projected
  arc A77 (-7.4111, 28.8847) -> (-7.777, 29.9735) centre (-13.5311, 27.4336) ccw projected
  arc A78 (-7.777, 29.9735) -> (-8.8968, 31.9385) centre (-17.7315, 25.6027) ccw projected
  arc A79 (-8.8968, 31.9385) -> (-10.3249, 31.7581) centre (-6.228, 5.0707) ccw projected
  arc A80 (-10.3249, 31.7581) -> (-10.9208, 29.5763) centre (-0.1921, 27.8185) ccw projected
  arc A81 (-10.9208, 29.5763) -> (-11.0044, 28.4308) centre (-4.7158, 28.5472) ccw projected
  arc A82 (-11.0044, 28.4308) -> (-10.9735, 28.0788) centre (-8.7169, 28.4546) ccw projected
  line L20 (-10.9735, 28.0788) -> (-10.773, 27.1069) projected
  arc A83 (-10.773, 27.1069) -> (-12.8612, 26.5708) centre (-6.228, 5.0707) ccw projected
  line L21 (-12.8612, 26.5708) -> (-13.1538, 27.519) projected
  arc A84 (-13.1538, 27.519) -> (-13.2962, 27.8424) centre (-15.3122, 26.7612) ccw projected
  arc A85 (-13.2962, 27.8424) -> (-13.9214, 28.8059) centre (-18.8631, 24.9148) ccw projected
  arc A86 (-13.9214, 28.8059) -> (-15.4947, 30.4307) centre (-22.4762, 22.0969) ccw projected
  arc A87 (-15.4947, 30.4307) -> (-16.8331, 29.9008) centre (-6.228, 5.0707) ccw projected
  arc A88 (-16.8331, 29.9008) -> (-16.8676, 27.6394) centre (-6.0388, 28.6049) ccw projected
  arc A89 (-16.8676, 27.6394) -> (-16.6638, 26.509) centre (-10.6017, 28.1857) ccw projected
  arc A90 (-16.6638, 26.509) -> (-16.5463, 26.1758) centre (-14.4541, 27.101) ccw projected
  line L22 (-16.5463, 26.1758) -> (-16.1104, 25.2843) projected
  arc A91 (-16.1104, 25.2843) -> (-17.9997, 24.2457) centre (-6.228, 5.0707) ccw projected
  line L23 (-17.9997, 24.2457) -> (-18.5188, 25.0914) projected
  arc A92 (-18.5188, 25.0914) -> (-18.7372, 25.3692) centre (-20.421, 23.8206) ccw projected
  arc A93 (-18.7372, 25.3692) -> (-19.5824, 26.1469) centre (-23.4012, 21.1491) ccw projected
  arc A94 (-19.5824, 26.1469) -> (-21.5103, 27.3295) centre (-26.1999, 17.5212) ccw projected
  arc A95 (-21.5103, 27.3295) -> (-22.6749, 26.4834) centre (-6.228, 5.0707) ccw projected
  arc A96 (-22.6749, 26.4834) -> (-22.146, 24.2844) centre (-11.8975, 27.9126) ccw projected
  arc A97 (-22.146, 24.2844) -> (-21.6674, 23.2402) centre (-16.2127, 26.3719) ccw projected
  arc A98 (-21.6674, 23.2402) -> (-21.4707, 22.9467) centre (-19.6743, 24.3631) ccw projected
  line L24 (-21.4707, 22.9467) -> (-20.8269, 22.1916) projected
  arc A99 (-20.8269, 22.1916) -> (-22.3984, 20.7158) centre (-6.228, 5.0707) ccw projected
  line L25 (-22.3984, 20.7158) -> (-23.1116, 21.4058) projected
  arc A100 (-23.1116, 21.4058) -> (-23.3922, 21.6205) centre (-24.638, 19.7019) ccw projected
  arc A101 (-23.3922, 21.6205) -> (-24.4043, 22.1637) centre (-26.8602, 16.3732) ccw projected
  arc A102 (-24.4043, 22.1637) -> (-26.5657, 22.8296) centre (-28.6688, 12.1633) ccw projected
  arc A103 (-26.5657, 22.8296) -> (-27.4833, 21.7205) centre (-6.228, 5.0707) ccw projected
  arc A104 (-27.4833, 21.7205) -> (-26.4241, 19.7222) centre (-17.3999, 25.785) ccw projected
  arc A105 (-26.4241, 19.7222) -> (-25.7009, 18.8298) centre (-21.1964, 23.2196) ccw projected
  arc A106 (-25.7009, 18.8298) -> (-25.4374, 18.5944) centre (-24.0497, 20.4131) ccw projected
  line L26 (-25.4374, 18.5944) -> (-24.626, 18.0232) projected
  arc A107 (-24.626, 18.0232) -> (-25.7812, 16.2029) centre (-6.228, 5.0707) ccw projected
  line L27 (-25.7812, 16.2029) -> (-26.6435, 16.6938) projected
  arc A108 (-26.6435, 16.6938) -> (-26.9688, 16.832) centre (-27.6983, 14.6638) ccw projected
  arc A109 (-26.9688, 16.832) -> (-28.0841, 17.1064) centre (-29.0228, 10.8871) ccw projected
  arc A110 (-28.0841, 17.1064) -> (-30.3432, 17.2139) centre (-29.7276, 6.3596) ccw projected
  arc A111 (-30.3432, 17.2139) -> (-30.9561, 15.9115) centre (-6.228, 5.0707) ccw projected
  arc A112 (-30.9561, 15.9115) -> (-29.4333, 14.2393) centre (-22.2003, 22.3559) ccw projected
  arc A113 (-29.4333, 14.2393) -> (-28.5109, 13.5548) centre (-25.2396, 18.9269) ccw projected
  arc A114 (-28.5109, 13.5548) -> (-28.1971, 13.3923) centre (-27.3053, 15.499) ccw projected
  line L28 (-28.1971, 13.3923) -> (-27.2691, 13.0408) projected
  arc A115 (-27.2691, 13.0408) -> (-27.9353, 10.9904) centre (-6.228, 5.0707) ccw projected
  line L29 (-27.9353, 10.9904) -> (-28.8927, 11.2515) projected
  arc A116 (-28.8927, 11.2515) -> (-29.2421, 11.3045) centre (-29.4094, 9.023) ccw projected
  arc A117 (-29.2421, 11.3045) -> (-30.3906, 11.2929) centre (-29.7531, 5.0356) ccw projected
  arc A118 (-30.3906, 11.2929) -> (-32.6055, 10.8352) centre (-29.3099, 0.475) ccw projected
  arc A119 (-32.6055, 10.8352) -> (-32.8752, 9.4213) centre (-6.228, 5.0707) ccw projected
  arc A120 (-32.8752, 9.4213) -> (-30.9844, 8.1803) centre (-25.9972, 17.8407) ccw projected
  arc A121 (-30.9844, 8.1803) -> (-29.9207, 7.7468) centre (-28.0882, 13.7636) ccw projected
  arc A122 (-29.9207, 7.7468) -> (-29.5764, 7.6674) centre (-29.2365, 9.9297) ccw projected
  line L30 (-29.5764, 7.6674) -> (-28.5902, 7.5577) projected
  arc A123 (-28.5902, 7.5577) -> (-28.7255, 5.4061) centre (-6.228, 5.0707) ccw projected
  line L31 (-28.7255, 5.4061) -> (-29.7177, 5.4209) projected
  arc A124 (-29.7177, 5.4209) -> (-30.0693, 5.3853) centre (-29.664, 3.1339) ccw projected
  arc A125 (-30.0693, 5.3853) -> (-31.1789, 5.0885) centre (-29.0053, -0.8138) ccw projected
  arc A126 (-31.1789, 5.0885) -> (-33.2104, 4.0943) centre (-27.4418, -5.1208) ccw projected
  arc A127 (-33.2104, 4.0943) -> (-33.12, 2.6577) centre (-6.228, 5.0707) ccw projected
  arc A128 (-33.12, 2.6577) -> (-30.9799, 1.926) centre (-28.5519, 12.5231) ccw projected
  arc A129 (-30.9799, 1.926) -> (-29.8419, 1.7705) centre (-29.5632, 8.0541) ccw projected
  arc A130 (-29.8419, 1.7705) -> (-29.4886, 1.7793) centre (-29.722, 4.055) ccw projected
  line L32 (-29.4886, 1.7793) -> (-28.5061, 1.9184) projected
  arc A131 (-28.5061, 1.9184) -> (-28.1021, -0.1994) centre (-6.228, 5.0707) ccw projected
  line L33 (-28.1021, -0.1994) -> (-29.0668, -0.4318) projected
  arc A132 (-29.0668, -0.4318) -> (-29.3985, -0.5536) centre (-28.4461, -2.6336) ccw projected
  arc A133 (-29.3985, -0.5536) -> (-30.3994, -1.1171) centre (-26.8263, -6.2934) ccw projected
  arc A134 (-30.3994, -1.1171) -> (-32.1198, -2.5852) centre (-24.2408, -10.0763) ccw projected
  arc A135 (-32.1198, -2.5852) -> (-31.675, -3.9543) centre (-6.228, 5.0707) ccw projected
  arc A136 (-31.675, -3.9543) -> (-29.4202, -4.1308) centre (-29.7038, 6.7373) ccw projected
  arc A137 (-29.4202, -4.1308) -> (-28.2793, -3.9983) centre (-29.572, 2.1572) ccw projected
  arc A138 (-28.2793, -3.9983) -> (-27.9393, -3.9019) centre (-28.7313, -1.7558) ccw projected
  line L34 (-27.9393, -3.9019) -> (-27.0222, -3.5229) projected
  arc A139 (-27.0222, -3.5229) -> (-26.1043, -5.4737) centre (-6.228, 5.0707) ccw projected
  line L35 (-26.1043, -5.4737) -> (-26.9809, -5.9387) projected
  arc A140 (-26.9809, -5.9387) -> (-27.2718, -6.1392) centre (-25.8321, -7.9169) ccw projected
  arc A141 (-27.2718, -6.1392) -> (-28.1012, -6.9339) centre (-23.353, -11.0589) ccw projected
  arc A142 (-28.1012, -6.9339) -> (-29.4024, -8.7837) centre (-19.908, -14.08) ccw projected
  arc A143 (-29.4024, -8.7837) -> (-28.6311, -9.9991) centre (-6.228, 5.0707) ccw projected
  arc A144 (-28.6311, -9.9991) -> (-26.4033, -9.6093) centre (-29.3808, 0.8467) ccw projected
  arc A145 (-26.4033, -9.6093) -> (-25.3311, -9.1973) centre (-28.1141, -3.5567) ccw projected
  arc A146 (-25.3311, -9.1973) -> (-25.0258, -9.0194) centre (-26.3266, -7.1376) ccw projected
  line L36 (-25.0258, -9.0194) -> (-24.2318, -8.4242) projected
  arc A147 (-24.2318, -8.4242) -> (-22.8576, -10.0854) centre (-6.228, 5.0707) ccw projected
  line L37 (-22.8576, -10.0854) -> (-23.591, -10.7538) projected
  arc A148 (-23.591, -10.7538) -> (-23.8229, -11.0204) centre (-21.9863, -12.3842) ccw projected
  arc A149 (-23.8229, -11.0204) -> (-24.4285, -11.9964) centre (-18.8037, -14.811) ccw projected
  arc A150 (-24.4285, -11.9964) -> (-25.2289, -14.1117) centre (-14.7156, -16.8804) ccw projected
  arc A151 (-25.2289, -14.1117) -> (-24.1796, -15.0971) centre (-6.228, 5.0707) ccw projected
  arc A152 (-24.1796, -15.0971) -> (-22.1186, -14.1655) centre (-27.6029, -4.7784) ccw projected
  arc A153 (-22.1186, -14.1655) -> (-21.1826, -13.4998) centre (-25.2809, -8.7285) ccw projected
  arc A154 (-21.1826, -13.4998) -> (-20.9312, -13.2516) centre (-22.6591, -11.7524) ccw projected
  line L38 (-20.9312, -13.2516) -> (-20.3101, -12.4776) projected
  arc A155 (-20.3101, -12.4776) -> (-18.5659, -13.7448) centre (-6.228, 5.0707) ccw projected
  line L39 (-18.5659, -13.7448) -> (-19.1101, -14.5747) projected
  arc A156 (-19.1101, -14.5747) -> (-19.2684, -14.8906) centre (-17.1503, -15.7548) ccw projected
  arc A157 (-19.2684, -14.8906) -> (-19.6123, -15.9865) centre (-13.4642, -17.3138) ccw projected
  arc A158 (-19.6123, -15.9865) -> (-19.8615, -18.2344) centre (-8.9899, -18.3015) ccw projected
  arc A159 (-19.8615, -18.2344) -> (-18.6, -18.9279) centre (-6.228, 5.0707) ccw projected
  arc A160 (-18.6, -18.9279) -> (-16.8356, -17.513) centre (-24.482, -9.7847) ccw projected
  arc A161 (-16.8356, -17.513) -> (-16.0945, -16.6354) centre (-21.2506, -13.0332) ccw projected
  arc A162 (-16.0945, -16.6354) -> (-15.9127, -16.3325) centre (-17.9591, -15.3101) ccw projected
  line L40 (-15.9127, -16.3325) -> (-15.5036, -15.4284) projected
  arc A163 (-15.5036, -15.4284) -> (-13.4991, -16.222) centre (-6.228, 5.0707) ccw projected
  line L41 (-13.4991, -16.222) -> (-13.8197, -17.1611) projected
  arc A164 (-13.8197, -17.1611) -> (-13.8946, -17.5064) centre (-11.6281, -17.8168) ccw projected
  arc A165 (-13.8946, -17.5064) -> (-13.9551, -18.6534) centre (-7.6701, -18.4101) ccw projected
  arc A166 (-13.9551, -18.6534) -> (-13.6374, -20.8927) centre (-3.0907, -18.2541) ccw projected
  arc A167 (-13.6374, -20.8927) -> (-12.2431, -21.2507) centre (-6.228, 5.0707) ccw projected
  arc A168 (-12.2431, -21.2507) -> (-10.8859, -19.4415) centre (-20.2141, -13.8576) ccw projected
  arc A169 (-10.8859, -19.4415) -> (-10.3864, -18.4072) centre (-16.2763, -16.2004) ccw projected
  arc A170 (-10.3864, -18.4072) -> (-10.2856, -18.0685) centre (-12.5221, -17.5872) ccw projected
  line L42 (-10.2856, -18.0685) -> (-10.1142, -17.0911) projected
  arc A171 (-10.1142, -17.0911) -> (-7.9753, -17.3613) centre (-6.228, 5.0707) ccw projected
  line L43 (-7.9753, -17.3613) -> (-8.0524, -18.3506) projected
  arc A172 (-8.0524, -18.3506) -> (-8.039, -18.7037) centre (-5.7665, -18.4406) ccw projected
  arc A173 (-8.039, -18.7037) -> (-7.8124, -19.8298) centre (-1.7853, -18.0311) ccw projected
  arc A174 (-7.8124, -19.8298) -> (-6.9478, -21.9197) centre (2.6114, -16.7411) ccw projected
  arc A175 (-6.9478, -21.9197) -> (-5.5083, -21.9197) centre (-6.228, 5.0707) ccw projected
  arc A176 (-5.5083, -21.9197) -> (-4.6437, -19.8298) centre (-15.0674, -16.7411) ccw projected
  arc A177 (-4.6437, -19.8298) -> (-4.4171, -18.7037) centre (-10.6707, -18.0311) ccw projected
  arc A178 (-4.4171, -18.7037) -> (-4.4037, -18.3506) centre (-6.6895, -18.4406) ccw projected
  line L44 (-4.4037, -18.3506) -> (-4.4807, -17.3613) projected
  arc A179 (-4.4807, -17.3613) -> (-2.3418, -17.0911) centre (-6.228, 5.0707) ccw projected
  line L45 (-2.3418, -17.0911) -> (-2.1704, -18.0685) projected
  arc A180 (-2.1704, -18.0685) -> (-2.0696, -18.4072) centre (0.066, -17.5872) ccw projected
  arc A181 (-2.0696, -18.4072) -> (-1.5701, -19.4415) centre (3.8203, -16.2004) ccw projected
  arc A182 (-1.5701, -19.4415) -> (-0.2129, -21.2507) centre (7.758, -13.8576) ccw projected
  arc A183 (-0.2129, -21.2507) -> (1.1813, -20.8927) centre (-6.228, 5.0707) ccw projected
  arc A184 (1.1813, -20.8927) -> (1.4991, -18.6534) centre (-9.3653, -18.2541) ccw projected
  arc A185 (1.4991, -18.6534) -> (1.4385, -17.5064) centre (-4.786, -18.4101) ccw projected
  arc A186 (1.4385, -17.5064) -> (1.3637, -17.1611) centre (-0.828, -17.8168) ccw projected
  line L46 (1.3637, -17.1611) -> (1.043, -16.222) projected
  arc A187 (1.043, -16.222) -> (3.0475, -15.4284) centre (-6.228, 5.0707) ccw projected
  line L47 (3.0475, -15.4284) -> (3.4566, -16.3325) projected
  arc A188 (3.4566, -16.3325) -> (3.6385, -16.6354) centre (5.5031, -15.3101) ccw projected
  arc A189 (3.6385, -16.6354) -> (4.3795, -17.513) centre (8.7945, -13.0332) ccw projected
  arc A190 (4.3795, -17.513) -> (6.144, -18.9279) centre (12.0259, -9.7847) ccw projected
  arc A191 (6.144, -18.9279) -> (7.4054, -18.2344) centre (-6.228, 5.0707) ccw projected
  arc A192 (7.4054, -18.2344) -> (7.1563, -15.9865) centre (-3.4661, -18.3015) ccw projected
  arc A193 (7.1563, -15.9865) -> (6.8124, -14.8906) centre (1.0082, -17.3138) ccw projected
  arc A194 (6.8124, -14.8906) -> (6.654, -14.5747) centre (4.6943, -15.7548) ccw projected
  line L48 (6.654, -14.5747) -> (6.1099, -13.7448) projected
  arc A195 (6.1099, -13.7448) -> (7.854, -12.4776) centre (-6.228, 5.0707) ccw projected
  line L49 (7.854, -12.4776) -> (8.4751, -13.2516) projected
  arc A196 (8.4751, -13.2516) -> (8.7266, -13.4998) centre (10.203, -11.7524) ccw projected
  arc A197 (8.7266, -13.4998) -> (9.6626, -14.1655) centre (12.8248, -8.7285) ccw projected
  arc A198 (9.6626, -14.1655) -> (11.7235, -15.0971) centre (15.1468, -4.7784) ccw projected
  arc A199 (11.7235, -15.0971) -> (12.7728, -14.1117) centre (-6.228, 5.0707) ccw projected
  circle A200 centre (-6.228, 7.8707) radius 1.5 projected
  circle A201 centre (-9.028, 5.0707) radius 1.5 projected
  circle A202 centre (-6.228, 2.2707) radius 1.5 projected
  circle A203 centre (-3.428, 5.0707) radius 1.5 projected
  circle A204 centre (-6.228, 5.0707) radius 22.5
  arc A205 (16.2695, 5.4061) -> (16.1341, 7.5577) centre (-6.228, 5.0707) ccw projected
  circle A206 centre (-6.228, 5.0707) radius 4.3
  arc A207 (15.6461, -0.1994) -> (16.05, 1.9184) centre (-6.228, 5.0707) ccw projected
  circle A208 centre (-6.228, 5.0707) radius 19.5
  circle A209 centre (-6.228, 5.0707) radius 7.3
  line L50 (-6.228, 5.0707) -> (-6.228, 24.5707) construction
  line L51 (-7.728, 24.513) -> (-8.728, 11.9293)
  line L52 (-4.728, 24.513) -> (-3.728, 11.9293)
  line L53 (-25.6703, 6.5707) -> (-13.0866, 7.5707)
  line L54 (-25.6703, 3.5707) -> (-13.0866, 2.5707)
  line L55 (-7.728, -14.3715) -> (-8.728, -1.7878)
  line L56 (-4.728, -14.3715) -> (-3.728, -1.7878)
  line L57 (13.2142, 3.5707) -> (0.6305, 2.5707)
  line L58 (13.2142, 6.5707) -> (0.6305, 7.5707)
  point P0 (0, 0)
  dimension "d19" = 3
  dimension "d20" = 3
  dimension "d21" = 1.5
  dimension "d22" = 2.5
  dimension "d25" = 360
  constraints: 18 end point, 3 centre point, 3 tangent, 2 coincident, 2 point on circle, 2 symmetric about line, 1 vertical, 28 other
  measures "d19" radial gap between concentric circles of A204 A208
  measures "d21" distance from line of L50 L51.start
  measures "d22" distance from line of L50 L51.end
extrude "押し出し2" cut sketch "スケッチ2" against normal blind 10 contours L58 A209 L52 A208 | A208 L56 A209 L57 | L51 A209 L53 A208 | A208 L54 A209 L55
fillet "フィレット1" radius 1.05 16 edges at (-25.6703, 6.5707, 2) (-7.728, 24.513, 2) (-8.728, 11.9293, 2) (-13.0866, 7.5707, 2) (-13.0866, 2.5707, 2) (-8.728, -1.7878, 2) (-25.6703, 3.5707, 2) (-7.728, -14.3715, 2) (-3.728, -1.7878, 2) (0.6305, 2.5707, 2) (13.2142, 3.5707, 2) (-4.728, -14.3715, 2) (0.6305, 7.5707, 2) (-3.728, 11.9293, 2) (-4.728, 24.513, 2) (13.2142, 6.5707, 2)
sketch "スケッチ3" plane through (0, 0, 4) normal (0, 0, 1) x (1, 0, 0)
  arc A0 (0.4014, 8.1269) -> (-3.1719, 11.7002) centre (-6.228, 5.0707) ccw projected
  circle A1 centre (-6.228, 5.0707) radius 9.025
  point P0 (0, 0)
  dimension "d30" = 18.05
  constraints: 1 centre point, 1 coincident
  measures "d30" diameter of A1
extrude "押し出し3" cut sketch "スケッチ3" against normal blind 0.5
